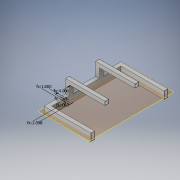
# Autodesk Inventor part: ShooterFrame
Saved by Autodesk Inventor 2016 SP1 (Build 200210100, 210)
## iProperties
Created: 2016-01-24
Part Number: ShooterFrame
Material: Generic
Document SubType Name: Modeling
Designer: steele
Density: 1 g/cm^3
Appearance: Default
Author: steele
Autodesk Inventor part; units mm, degrees
sketch "Sketch10" plane through (0, 0, 0) normal (0, 1, 0) x (-1, 0, 0)
  line L0 (0, 0) -> (0, 247.65)
  line L1 (0, 247.65) -> (-304.8, 247.65)
  line L2 (0, 0) -> (-304.8, 0) construction
  line L3 (0, 0) -> (0, -247.65)
  line L4 (0, -247.65) -> (-304.8, -247.65)
  dimension "d31" = 247.65
  dimension "d32" = 304.8
  constraints: 10 end point, 2 symmetric about line, 1 horizontal, 1 perpendicular, 1 vertical
  measures "d31" distance of L0.start L0.end
  measures "d32" distance of L0.end L1.end
ref_plane "Work Plane2" through (304.8, 0, 0) normal (1, 0, 0) x (0, 1, 0)
sketch "Sketch11" plane through (304.8, 0, 0) normal (1, 0, 0) x (0, 1, 0)
  line L0 (-25.4, 260.35) -> (-25.4, 234.95)
  line L1 (-25.4, 234.95) -> (25.4, 234.95)
  line L2 (25.4, 234.95) -> (25.4, 260.35)
  line L3 (25.4, 260.35) -> (-25.4, 260.35)
  line L4 (-25.4, 260.35) -> (25.4, 234.95) construction
  line L5 (-25.4, 234.95) -> (25.4, 260.35) construction
  line L6 (-22.225, 257.175) -> (-22.225, 238.125)
  line L7 (-22.225, 238.125) -> (22.225, 238.125)
  line L8 (22.225, 238.125) -> (22.225, 257.175)
  line L9 (22.225, 257.175) -> (-22.225, 257.175)
  line L10 (-22.225, 257.175) -> (22.225, 238.125) construction
  line L11 (-22.225, 238.125) -> (22.225, 257.175) construction
  point P0 (0, 0)
  point P1 (0, 247.65)
  dimension "d34" = 247.65
  dimension "d35" = 25.4
  dimension "d36" = 50.8
  dimension "d37" = 3.175
  dimension "d38" = 3.175
  constraints: 24 end point, 4 midpoint, 4 parallel, 2 perpendicular, 2 vertical
  measures "d34" distance of point (0, 0) point (0, 247.65)
  measures "d35" distance of L1.end L2.end
  measures "d36" distance of L2.end L0.start
  measures "d37" distance between parallel lines of L3 L9
  measures "d38" distance between parallel lines of L0 L6
sweep "Sweep5" add profiles "Sketch11" path "Sketch10" path curves L1 L0 L3 L4
sketch "Sketch12" plane through (304.8, 25.4, 260.35) normal (0, 1, 0) x (1, 0, 0)
  line L0 (-304.8, 260.35) -> (-304.8, 0) construction
  line L1 (0, 0) -> (-317.5, 0) construction
  line L2 (-317.5, 146.05) -> (-292.1, 146.05)
  line L3 (-292.1, 146.05) -> (-292.1, 171.45)
  line L4 (-292.1, 171.45) -> (-317.5, 171.45)
  line L5 (-317.5, 171.45) -> (-317.5, 146.05)
  line L6 (-317.5, 146.05) -> (-292.1, 171.45) construction
  line L7 (-292.1, 146.05) -> (-317.5, 171.45) construction
  line L8 (-295.275, 22.225) -> (-295.275, 498.475) projected
  line L9 (-315.9125, 147.6375) -> (-293.6875, 147.6375)
  line L10 (-293.6875, 147.6375) -> (-293.6875, 169.8625)
  line L11 (-293.6875, 169.8625) -> (-315.9125, 169.8625)
  line L12 (-315.9125, 169.8625) -> (-315.9125, 147.6375)
  line L13 (-315.9125, 147.6375) -> (-293.6875, 169.8625) construction
  line L14 (-293.6875, 147.6375) -> (-315.9125, 169.8625) construction
  point P0 (-304.8, 158.75)
  dimension "d41" = 25.4
  dimension "d42" = 25.4
  dimension "d43" = 101.6
  dimension "d44" = 1.5875
  dimension "d45" = 1.5875
  constraints: 26 end point, 4 midpoint, 4 parallel, 4 perpendicular, 2 point on line, 1 vertical
  measures "d41" distance of L4.end L2.start
  measures "d42" distance of L2.start L2.end
  measures "d43" distance of point (-304.8, 158.75) L0.start
  measures "d44" distance between parallel lines of L5 L12
  measures "d45" distance between parallel lines of L2 L9
ref_plane "Work Plane3" through (0, 0, 76.2) normal (0, 0, 1) x (1, 0, 0)
sketch "Sketch13" plane through (0, 0, 76.2) normal (0, 0, 1) x (1, 0, 0)
  line L0 (304.8, 25.4) -> (-12.7, 25.4) projected
  line L1 (0, 25.4) -> (0, 101.6)
  line L2 (0, 101.6) -> (254, 101.6)
  point P0 (0, 0)
  dimension "d47" = 254
  dimension "d48" = 76.2
  constraints: 4 end point, 1 perpendicular, 1 point on line, 1 vertical
  measures "d47" distance of L1.end L2.end
  measures "d48" distance of L1.start L1.end
sweep "Sweep6" add profiles "Sketch12" path "Sketch13" path curves L1 L2 contours L5 L4 L8 L11 L12 L9 L2 | L8 L9 L10 L11 L4 L3 L2
mirror "Mirror2" about plane through (0, 0, 0) normal (0, 0, 1) of "Sweep6"
sketch "Sketch14" plane through (304.8, -25.4, 234.95) normal (0, -1, 0) x (1, 0, 0)
  line L0 (-304.8, -234.95) -> (-304.8, 22.225) construction
  line L1 (0, 22.225) -> (-314.325, 22.225) construction
  line L2 (-317.5, -120.65) -> (-317.5, -146.05)
  line L3 (-317.5, -146.05) -> (-292.1, -146.05)
  line L4 (-292.1, -146.05) -> (-292.1, -120.65)
  line L5 (-292.1, -120.65) -> (-317.5, -120.65)
  line L6 (-317.5, -120.65) -> (-292.1, -146.05) construction
  line L7 (-317.5, -146.05) -> (-292.1, -120.65) construction
  line L8 (-315.9125, -122.2375) -> (-315.9125, -144.4625)
  line L9 (-315.9125, -144.4625) -> (-293.6875, -144.4625)
  line L10 (-293.6875, -144.4625) -> (-293.6875, -122.2375)
  line L11 (-293.6875, -122.2375) -> (-315.9125, -122.2375)
  line L12 (-315.9125, -122.2375) -> (-293.6875, -144.4625) construction
  line L13 (-315.9125, -144.4625) -> (-293.6875, -122.2375) construction
  line L14 (-317.5, 25.4) -> (-317.5, -495.3) projected
  point P0 (-304.8, -133.35)
  dimension "d52" = 101.6
  dimension "d53" = 25.4
  dimension "d54" = 25.4
  dimension "d55" = 1.5875
  dimension "d56" = 1.5875
  constraints: 26 end point, 5 parallel, 4 midpoint, 2 perpendicular, 2 point on line, 1 vertical
  measures "d52" distance of point (-304.8, -133.35) L0.start
  measures "d53" distance of L4.end L2.start
  measures "d54" distance of L2.start L2.end
  measures "d55" distance between parallel lines of L5 L11
  measures "d56" distance between parallel lines of L8 L14
equation "\"d31\" = halfOfWidth"
equation "\"d32\" = length"
equation "\"d34\" = halfOfWidth"
equation "\"d35\" = largeTubingWidth"
equation "\"d36\" = largeTubingHeight"
equation "\"d37\" = largeTubeThickness"
equation "\"d38\" = largeTubeThickness"
equation "\"d41\" = smallSupportTubeWidth"
equation "\"d42\" = smallSupportTubeWidth"
equation "\"d43\" = distaceToMiddleSmallSupportTube"
equation "\"d44\" = smallSupportTubeThickness"
equation "\"d45\" = smallSupportTubeThickness"
equation "\"d47\" = smallSupportTubeExtension"
equation "\"d48\" = smallSupportTubeLength"
equation "\"d52\" = distaceToMiddleSmallSupportTube"
equation "\"d53\" = smallSupportTubeWidth"
equation "\"d54\" = smallSupportTubeHeight"
equation "\"d55\" = smallSupportTubeThickness"
equation "\"d56\" = smallSupportTubeThickness"
equation "\"halfOfWidth\" = 247.65"
equation "\"length\" = 304.8"
equation "\"height\" = 241.3"
equation "\"largeTubingWidth\" = 25.4"
equation "\"largeTubingHeight\" = 50.8"
equation "\"largeTubeThickness\" = 3.175"
equation "\"d33\" = length"
equation "\"width\" = 508"
equation "\"smallSupportTubeWidth\" = 25.4"
equation "\"smallSupportTubeHeight\" = 25.4"
equation "\"smallSupportTubeThickness\" = 1.5875"
equation "\"distaceToMiddleSmallSupportTube\" = 101.6"
equation "\"smallSupportTubeLength\" = 76.2"
equation "\"d46\" = smallSupportTubeLength"
equation "\"smallSupportTubeExtension\" = 254"
body "Solid5"
